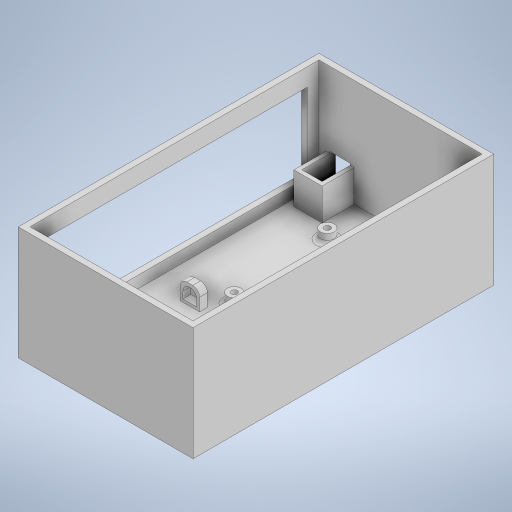
# Autodesk Inventor part: CajaControladora
Saved by Autodesk Inventor 2024 (Build 280153000, 153)
## iProperties
Created: 2023-11-26
Part Number: CajaControladora
Material: Genérico
Document SubType Name: Modeling
Designer: sergi
Density: 1 g/cm^3
Appearance: Valor por defecto
Author: sergi
Autodesk Inventor part; units mm, degrees
ref_plane "YZ Plane" through (0, 0, 0) normal (1, 0, 0) x (0, 1, 0)
ref_plane "XZ Plane" through (0, 0, 0) normal (0, 1, 0) x (-1, 0, 0)
ref_plane "XY Plane" through (0, 0, 0) normal (0, 0, 1) x (1, 0, 0)
sketch "Arduino" plane through (0, 0, 0) normal (0, 1, 0) x (-1, 0, 0)
  line L0 (14.7, 0) -> (48.2, 0)
  line L1 (53.2, -2.5) -> (53.2, -68.5)
  line L2 (0, -2.5) -> (12.2, -2.5)
  line L3 (12.2, -2.5) -> (14.7, 0)
  line L4 (53.2, -2.5) -> (50.7, -2.5)
  line L5 (50.7, -2.5) -> (48.2, 0)
  line L6 (0, -2.5) -> (0, -68.5)
  line L7 (0, -68.5) -> (9.8, -68.5)
  line L8 (9.8, -68.5) -> (9.8, -76.7)
  line L9 (9.8, -76.7) -> (21.92, -76.7)
  line L10 (21.92, -76.7) -> (21.92, -68.5)
  line L11 (21.92, -68.5) -> (41.57, -68.5)
  line L12 (41.57, -68.5) -> (41.57, -73.55)
  line L13 (41.57, -73.55) -> (50.62, -73.55)
  line L14 (50.62, -73.55) -> (50.62, -68.5)
  line L15 (53.2, -68.5) -> (50.62, -68.5)
  line L16 (0, -68.5) -> (9.8, -68.5)
  line L17 (21.92, -68.5) -> (41.57, -68.5)
  line L18 (50.62, -68.5) -> (53.2, -68.5)
  line L19 (0, -2.5) -> (12.2, -2.5)
  line L20 (50.7, -2.5) -> (53.2, -2.5)
  circle A0 centre (18, -2.25) radius 1.575
  circle A1 centre (46.2, -2.25) radius 1.575
  line L21 (53.2, -68.5) -> (53.2, -53.35)
  circle A2 centre (50.88, -54.5) radius 1.575
  circle A3 centre (2.3, -53.5) radius 1.575
  dimension "d4" = 135
  dimension "d5" = 2.5
  dimension "d6" = 135
  dimension "d7" = 66
  dimension "d8" = 9.8
  dimension "d9" = 12.12
  dimension "d10" = 19.65
  dimension "d11" = 5.05
  dimension "d12" = 9.05
  dimension "d15" = 3.15
  dimension "d17" = 3.15
  dimension "d21" = 3.15
  constraints: 44 end point, 15 perpendicular, 4 centre point, 1 horizontal, 1 point on line
  measures "d4" angle of L3 L2
  measures "d5" distance of L1.start L4.end
  measures "d6" angle of L4 L5
  measures "d7" distance of L6.end L2.start
  measures "d8" distance of L6.end L7.end
  measures "d9" distance of L8.end L9.end
  measures "d10" distance of L10.end L11.end
  measures "d11" distance of L11.end L12.end
  measures "d12" distance of L12.end L13.end
  measures "d15" diameter of A0
  measures "d17" diameter of A1
  measures "d21" diameter of A2
sketch "Conector" plane through (0, 0, 0) normal (0, 1, 0) x (-1, 0, 0)
  line L0 (21.92, -68.5) -> (41.57, -68.5) projected
  line L1 (41.57, -73.55) -> (50.62, -73.55) projected
  line L2 (53.2, -2.5) -> (53.2, -68.5) projected
  line L3 (0, -2.5) -> (0, -68.5) projected
  line L4 (0, -68.5) -> (9.8, -68.5) projected
  circle A0 centre (50.88, -54.5) radius 1.575 projected
  line L5 (53.2, -68.5) -> (50.62, -68.5) projected
  line L6 (50.62, -68.5) -> (53.2, -68.5) projected
  line L7 (53.2, -68.5) -> (53.2, -53.35) projected
  line L8 (50.62, -73.55) -> (50.62, -68.5) projected
  circle A1 centre (2.3, -53.5) radius 1.575 projected
  line L9 (21.92, -68.5) -> (41.57, -68.5) projected
  line L10 (0, -68.5) -> (9.8, -68.5) projected
  line L11 (21.92, -76.7) -> (21.92, -68.5) projected
  line L12 (9.8, -68.5) -> (9.8, -76.7) projected
  line L13 (9.8, -76.7) -> (21.92, -76.7) projected
  line L14 (41.57, -68.5) -> (41.57, -73.55) projected
  line L15 (61.92, -76.7) -> (71.32, -76.7)
  line L16 (71.32, -76.7) -> (71.32, -62.9)
  line L17 (71.32, -62.9) -> (61.92, -62.9)
  line L18 (61.92, -62.9) -> (61.92, -76.7)
  point P0 (0, 0)
  dimension "d25" = 40
  dimension "d26" = 9.4
  dimension "d27" = 13.8
  dimension "d28" = 11.3
  constraints: 8 end point, 2 parallel, 1 horizontal, 1 perpendicular
  measures "d25" distance of L11.start L15.start
  measures "d26" distance of L17.end L16.end
  measures "d27" distance of L16.end L15.end
  measures "d28" distance between parallel lines of L8 L18
sketch "PlacaRele" plane through (0, 0, 0) normal (0, 1, 0) x (-1, 0, 0)
  line L0 (0, 0) -> (0, 35)
  line L1 (0, 35) -> (70, 35)
  line L2 (70, 35) -> (70, 65)
  line L3 (70, 65) -> (0, 65)
  line L4 (0, 65) -> (0, 35)
  line L5 (69, 36) -> (1, 36)
  line L6 (1, 36) -> (1, 64)
  line L7 (1, 64) -> (69, 64)
  line L8 (69, 64) -> (69, 36)
  circle A0 centre (2, 37) radius 1
  circle A1 centre (2, 63) radius 1
  circle A2 centre (68, 37) radius 1
  circle A3 centre (68, 63) radius 1
  dimension "d29" = 35
  dimension "d30" = 70
  dimension "d31" = 30
  dimension "d32" = 1
  dimension "d34" = 2
  dimension "d35" = 2
  dimension "d36" = 2
  dimension "d37" = 2
  constraints: 18 end point, 8 tangent, 4 centre point, 4 parallel, 2 perpendicular, 1 horizontal, 1 vertical, 3 other
  measures "d29" distance of L0.start L0.end
  measures "d30" distance of L3.end L2.end
  measures "d31" distance of L2.end L1.end
  measures "d32" distance between parallel lines of L1 L5
  measures "d34" diameter of A0
  measures "d35" diameter of A1
  measures "d36" diameter of A2
  measures "d37" diameter of A3
sketch "Boceto4" plane through (0, 0, 0) normal (0, 1, 0) x (-1, 0, 0)
  line L0 (0, 65) -> (71.32, 65)
  line L1 (71.32, 65) -> (71.32, -76.7)
  line L2 (71.32, -76.7) -> (0, -76.7)
  line L3 (0, -76.7) -> (0, 65)
  line L4 (77.32, -76.7) -> (77.32, 71)
  line L5 (77.32, 71) -> (-6, 71)
  line L6 (-6, 71) -> (-6, -76.7)
  line L7 (80.32, 74) -> (80.32, -76.7)
  line L8 (-9, -76.7) -> (-9, 74)
  line L9 (-9, 74) -> (80.32, 74)
  line L10 (71.32, -62.9) -> (61.92, -62.9)
  line L11 (61.92, -62.9) -> (61.92, -76.7)
  line L12 (61.92, -76.7) -> (71.32, -76.7)
  line L13 (71.32, -76.7) -> (71.32, -62.9)
  line L14 (61.42, -62.4) -> (71.82, -62.4)
  line L15 (71.82, -62.4) -> (71.82, -76.7)
  line L16 (61.42, -76.7) -> (61.42, -62.4)
  line L17 (73.82, -60.4) -> (59.42, -60.4)
  line L18 (59.42, -60.4) -> (59.42, -76.7)
  line L19 (73.82, -76.7) -> (73.82, -60.4)
  line L20 (0, -76.7) -> (-6, -76.7)
  line L21 (71.32, -76.7) -> (77.32, -76.7)
  line L22 (80.32, -76.7) -> (80.32, -79.7)
  line L23 (80.32, -79.7) -> (-9, -79.7)
  line L24 (-9, -79.7) -> (-9, -76.7)
  line L25 (14.7, 0) -> (48.2, 0) projected
  line L26 (53.2, -2.5) -> (53.2, -68.5) projected
  line L27 (0, -2.5) -> (12.2, -2.5) projected
  line L28 (12.2, -2.5) -> (14.7, 0) projected
  line L29 (53.2, -2.5) -> (50.7, -2.5) projected
  line L30 (50.7, -2.5) -> (48.2, 0) projected
  line L31 (0, -2.5) -> (0, -68.5) projected
  line L32 (0, -2.5) -> (12.2, -2.5) projected
  circle A0 centre (18, -2.25) radius 1.575 projected
  circle A1 centre (46.2, -2.25) radius 1.575 projected
  line L33 (50.7, -2.5) -> (53.2, -2.5) projected
  line L34 (0, -68.5) -> (9.8, -68.5) projected
  circle A2 centre (50.88, -54.5) radius 1.575 projected
  line L35 (53.2, -68.5) -> (50.62, -68.5) projected
  line L36 (50.62, -68.5) -> (53.2, -68.5) projected
  line L37 (53.2, -68.5) -> (53.2, -53.35) projected
  line L38 (50.62, -73.55) -> (50.62, -68.5) projected
  line L39 (41.57, -73.55) -> (50.62, -73.55) projected
  circle A3 centre (2.3, -53.5) radius 1.575 projected
  line L40 (21.92, -68.5) -> (41.57, -68.5) projected
  line L41 (21.92, -68.5) -> (41.57, -68.5) projected
  line L42 (0, -68.5) -> (9.8, -68.5) projected
  line L43 (21.92, -76.7) -> (21.92, -68.5) projected
  line L44 (9.8, -68.5) -> (9.8, -76.7) projected
  line L45 (9.8, -76.7) -> (21.92, -76.7) projected
  line L46 (41.57, -68.5) -> (41.57, -73.55) projected
  line L47 (53.2, -68.5) -> (50.62, -68.5) projected
  line L48 (50.62, -68.5) -> (53.2, -68.5) projected
  line L49 (50.62, -73.55) -> (50.62, -68.5) projected
  line L50 (53.2, -68.5) -> (53.2, -53.35) projected
  circle A4 centre (50.88, -54.5) radius 1.575 projected
  line L51 (41.57, -73.55) -> (50.62, -73.55) projected
  line L52 (41.57, -68.5) -> (41.57, -73.55) projected
  line L53 (21.92, -68.5) -> (41.57, -68.5) projected
  line L54 (21.92, -76.7) -> (21.92, -68.5) projected
  line L55 (9.8, -68.5) -> (9.8, -76.7) projected
  line L56 (9.8, -76.7) -> (21.92, -76.7) projected
  line L57 (53.2, -2.5) -> (53.2, -68.5) projected
  line L58 (0, -68.5) -> (9.8, -68.5) projected
  line L59 (0, -68.5) -> (9.8, -68.5) projected
  circle A5 centre (2.3, -53.5) radius 1.575 projected
  line L60 (0, -2.5) -> (0, -68.5) projected
  line L61 (21.92, -68.5) -> (41.57, -68.5) projected
  point P0 (1, 64)
  point P1 (69, 36)
  point P2 (70, 35)
  point P3 (69, 64)
  point P4 (70, 65)
  point P5 (0, 0)
  point P6 (0, 0)
  dimension "d39" = 6
  dimension "d40" = 3
  dimension "d41" = 0.5
  dimension "d42" = 2
  dimension "d43" = 3
  constraints: 50 end point, 8 parallel, 8 perpendicular, 5 point on line, 3 horizontal, 1 vertical
  measures "d39" distance between parallel lines of L1 L4
  measures "d40" distance between parallel lines of L4 L7
  measures "d41" distance between parallel lines of L10 L14
  measures "d42" distance between parallel lines of L14 L17
  measures "d43" distance of L7.end L22.end
sketch "Boceto5" plane through (0, 0, 0) normal (0, 1, 0) x (-1, 0, 0)
  line L0 (-9, 74) -> (80.32, 74) projected
  line L1 (80.32, 74) -> (80.32, -76.7) projected
  line L2 (80.32, -79.7) -> (-9, -79.7) projected
  line L3 (-9, -76.7) -> (-9, 74) projected
  line L4 (-6, 71) -> (-6, -76.7) projected
  line L5 (71.32, -76.7) -> (0, -76.7) projected
  line L6 (0, -76.7) -> (-6, -76.7) projected
  line L7 (71.32, -76.7) -> (77.32, -76.7) projected
  line L8 (77.32, -76.7) -> (77.32, 71) projected
  line L9 (77.32, 71) -> (-6, 71) projected
  line L10 (80.32, -76.7) -> (80.32, -79.7) projected
  line L11 (-9, -79.7) -> (-9, -76.7) projected
  point P0 (0, 0)
extrude "Extrusión1" add sketch "Boceto5" along normal blind 50
sketch "Boceto6" plane through (0, 0, 0) normal (0, -1, 0) x (1, 0, 0)
  line L0 (9, 74) -> (9, -79.7) projected
  line L1 (-80.32, 74) -> (9, 74) projected
  line L2 (-80.32, -79.7) -> (-80.32, 74) projected
  line L3 (9, -79.7) -> (-80.32, -79.7) projected
  line L4 (-77.32, -76.7) -> (6, -76.7) projected
  line L5 (-77.32, 71) -> (-77.32, -76.7) projected
  line L6 (6, 71) -> (-77.32, 71) projected
  line L7 (6, -76.7) -> (6, 71) projected
  point P0 (0, 0)
extrude "Extrusión2" add sketch "Boceto6" along normal blind 5
sketch "Boceto7" plane through (0, -5, 0) normal (0, -1, 0) x (1, 0, 0)
  line L0 (-80.32, -79.7) -> (9, -79.7) projected
  line L1 (-80.32, 74) -> (-80.32, -79.7) projected
  line L2 (9, 74) -> (-80.32, 74) projected
  line L3 (9, -79.7) -> (9, 74) projected
  point P0 (0, 0)
extrude "Extrusión3" add sketch "Boceto7" along normal blind 3
sketch "Boceto10" plane through (-77.32, 50, -76.7) normal (0, 0, 1) x (1, 0, 0)
  line L0 (6, -50) -> (77.32, -50) projected
  line L1 (67.52, -50) -> (67.52, -48.4)
  line L2 (67.52, -48.4) -> (55.4, -48.4)
  line L3 (55.4, -48.4) -> (55.4, -37.7)
  line L4 (55.4, -37.7) -> (67.52, -37.7)
  line L5 (67.52, -37.7) -> (67.52, -48.4)
  line L6 (68.52, -36.7) -> (54.4, -36.7)
  line L7 (54.4, -36.7) -> (54.4, -49.4)
  line L8 (54.4, -49.4) -> (68.52, -49.4)
  line L9 (68.52, -49.4) -> (68.52, -36.7)
  point P0 (77.32, -50)
  point P1 (55.4, -50)
  point P2 (55.4, -50)
  point P3 (55.4, -50)
  point P4 (67.52, -50)
  dimension "d62" = 1.6
  dimension "d63" = 10.7
  dimension "d64" = 1
  constraints: 18 end point, 4 parallel, 2 perpendicular, 1 horizontal, 1 vertical, 4 other
  measures "d62" distance of L1.start L1.end
  measures "d63" distance of L2.end L3.end
  measures "d64" distance between parallel lines of L4 L6
extrude "Extrusión6" cut sketch "Boceto10" against normal blind 10.9 contours L2 L3 L4 L5 | L9 L8 L7 L6
sketch "Boceto8" plane through (0, -5, 0) normal (0, 1, 0) x (1, 0, 0)
  circle A0 centre (-2.3, 53.5) radius 1.575 projected
  circle A1 centre (-18, 2.25) radius 1.575 projected
  line L0 (-73.82, 60.4) -> (-59.42, 60.4) projected
  line L1 (-59.42, 60.4) -> (-59.42, 76.7) projected
  line L2 (-61.42, 62.4) -> (-71.82, 62.4) projected
  line L3 (-61.42, 76.7) -> (-61.42, 62.4) projected
  line L4 (-71.82, 62.4) -> (-71.82, 76.7) projected
  line L5 (-73.82, 76.7) -> (-73.82, 60.4) projected
  line L6 (0, -35) -> (-70, -35) projected
  line L7 (-70, -35) -> (-70, -65) projected
  line L8 (-70, -65) -> (0, -65) projected
  line L9 (0, -65) -> (0, -35) projected
  circle A2 centre (-2, -37) radius 1 projected
  circle A3 centre (-2, -63) radius 1 projected
  circle A4 centre (-68, -37) radius 1 projected
  circle A5 centre (-68, -63) radius 1 projected
  circle A6 centre (-46.2, 2.25) radius 1.575 projected
  circle A7 centre (-50.88, 54.5) radius 1.575 projected
  circle A8 centre (-2.3, 53.5) radius 3.575
  circle A9 centre (-18, 2.25) radius 3.575
  circle A10 centre (-46.2, 2.25) radius 3.575
  circle A11 centre (-50.88, 54.5) radius 3.575
  circle A12 centre (-68, -37) radius 2.5
  circle A13 centre (-68, -63) radius 2.5
  circle A14 centre (-2, -37) radius 2.5
  circle A15 centre (-2, -63) radius 2.5
  point P0 (0, 0)
  dimension "d50" = 2
  dimension "d51" = 2
  dimension "d52" = 2
  dimension "d53" = 2
  dimension "d54" = 1.5
  dimension "d55" = 1.5
  dimension "d56" = 1.5
  dimension "d57" = 1.5
  constraints: 8 centre point
  measures "d50" radial gap between concentric circles of A0 A8
  measures "d51" radial gap between concentric circles of A1 A9
  measures "d52" radial gap between concentric circles of A6 A10
  measures "d53" radial gap between concentric circles of A7 A11
  measures "d54" radial gap between concentric circles of A4 A12
  measures "d55" radial gap between concentric circles of A5 A13
  measures "d56" radial gap between concentric circles of A2 A14
  measures "d57" radial gap between concentric circles of A3 A15
extrude "Extrusión4" add sketch "Boceto8" along normal blind 5 contours A14 L9 L6 | L6 A14 | A14 L9 | A12 L7 L6 | L6 A12 | A15 L9 | L9 A15 L8 | L8 A15 | L7 A12 | A13 L8 | L8 A13 L7 | L7 A13 | A8 | A9 | A10 | A11 picked at (-1.9598, -35.3358) picked at (-67.9598, -35.3358) picked at (-1.9598, -64.6642) picked at (-67.9598, -64.6642)
sketch "Boceto9" plane through (0, -5, 0) normal (0, 1, 0) x (1, 0, 0)
  circle A0 centre (-68, -37) radius 2.5 projected
  circle A1 centre (-18, 2.25) radius 3.575 projected
  circle A2 centre (-46.2, 2.25) radius 3.575 projected
  circle A3 centre (-2, -37) radius 2.5 projected
  circle A4 centre (-68, -63) radius 2.5 projected
  circle A5 centre (-50.88, 54.5) radius 3.575 projected
  circle A6 centre (-2, -63) radius 2.5 projected
  circle A7 centre (-2.3, 53.5) radius 3.575 projected
  line L0 (-77.32, 76.7) -> (-77.32, -71) projected
  line L1 (-77.32, -71) -> (6, -71) projected
  line L2 (6, -71) -> (6, 76.7) projected
  line L3 (6, 76.7) -> (-77.32, 76.7) projected
  line L4 (-73.82, 76.7) -> (-73.82, 60.4) projected
  line L5 (-73.82, 60.4) -> (-59.42, 60.4) projected
  line L6 (-59.42, 60.4) -> (-59.42, 76.7) projected
  line L7 (-61.42, 76.7) -> (-61.42, 62.4) projected
  line L8 (-61.42, 62.4) -> (-71.82, 62.4) projected
  line L9 (-71.82, 62.4) -> (-71.82, 76.7) projected
  point P0 (0, 0)
sketch "Boceto11" plane through (-77.32, 50, -76.7) normal (0, 0, 1) x (1, 0, 0)
  line L0 (68.52, -49.4) -> (54.4, -49.4) projected
  line L1 (15.9, -50) -> (5.5, -50) projected
  line L2 (0, 0) -> (0, -55) projected
  line L3 (54.4, -49.4) -> (0, -49.4)
  line L4 (15.9, -50) -> (15.9, -49.4)
  line L5 (6, -50) -> (0, -50) projected
  line L6 (5.5, -50) -> (5.5, -49.4)
  line L7 (15.9, -49.4) -> (5.5, -49.4)
  line L8 (5.5, -49.4) -> (5.5, -37.7)
  line L9 (5.5, -37.7) -> (15.9, -37.7)
  line L10 (15.9, -37.7) -> (15.9, -49.4)
  point P0 (77.32, -50)
  point P1 (5.5, -50)
  dimension "d67" = 11.7
  constraints: 14 end point, 4 perpendicular, 4 point on line, 2 parallel, 1 horizontal
  measures "d67" distance of L7.end L8.end
extrude "Extrusión7" cut sketch "Boceto11" against normal blind 10.9 contours L3 L8 L9 L10
extrude "Extrusión8" add sketch "Boceto9" along normal up to surface (5.6 mm away) contours L3 L9 L8 L7 L6 L5 L4 | L3 L7 L8 L9
sketch "Boceto12" plane through (-71.82, 0.6, -79.7) normal (0, 1, 0) x (1, 0, 0)
  line L0 (12.4, -19.3) -> (12.4, -3) projected
  line L1 (-2, -19.3) -> (12.4, -19.3) projected
  line L2 (-2, -3) -> (-2, -19.3) projected
  line L3 (10.4, -3) -> (10.4, -17.3)
  line L4 (10.4, -17.3) -> (0, -17.3)
  line L5 (0, -17.3) -> (0, -3)
  line L6 (12.4, -3) -> (-2, -3)
  point P0 (71.82, -79.7)
  constraints: 8 end point, 1 perpendicular, 2 other
extrude "Extrusión9" add sketch "Boceto12" along normal blind 10.7 contours L1 L2 L6 L5 L4 L3 L0
sketch "Boceto13" plane through (0, 50, 0) normal (0, 1, 0) x (1, 0, 0)
  line L0 (9, -74) -> (9, 79.7) projected
  line L1 (9, 79.7) -> (-80.32, 79.7) projected
  line L2 (9, -74) -> (9, 79.7) projected
  line L3 (9, 79.7) -> (-80.32, 79.7) projected
  line L4 (-80.32, 79.7) -> (-80.32, -74) projected
  line L5 (-80.32, -74) -> (9, -74) projected
  line L6 (-77.32, 76.7) -> (6, 76.7) projected
  line L7 (6, 76.7) -> (6, -71) projected
  line L8 (6, -71) -> (-77.32, -71) projected
  line L9 (-77.32, -71) -> (-77.32, 76.7) projected
  line L10 (9, 79.7) -> (-71, 79.7)
  line L11 (-71, 79.7) -> (-71, -0.3)
  line L12 (-71, -0.3) -> (9, -0.3)
  line L13 (9, -0.3) -> (9, 79.7)
  point P0 (0, 0)
  dimension "d74" = 80
  dimension "d75" = 80
  constraints: 8 end point, 2 parallel, 1 horizontal, 1 perpendicular
  measures "d74" distance of L12.end L11.end
  measures "d75" distance of L11.end L10.end
fillet "Empalme1" radius 2 8 edges at (-5.875, -5, -53.5) (-21.575, -5, -2.25) (-49.775, -5, -2.25) (-54.455, -5, -54.5) (-4.5, -5, 37) (-70.5, -5, 37) (-70.5, -5, 63) (-4.5, -5, 63)
sketch "Boceto14" plane through (0, -5, 0) normal (0, 1, 0) x (1, 0, 0)
  circle A0 centre (-18, 2.25) radius 5.575 projected
  line L0 (-18, -3.325) -> (-18, -6.325)
  line L1 (-18, -6.325) -> (9.6696, -6.325)
  line L2 (9.6696, -6.325) -> (-86.9175, -6.325)
  line L3 (0, -35) -> (-70, -35) projected
  circle A1 centre (-68, -63) radius 4.5 projected
  circle A2 centre (-2, -37) radius 4.5 projected
  circle A3 centre (-46.2, 2.25) radius 5.575 projected
  circle A4 centre (-2.3, 53.5) radius 5.575 projected
  line L4 (-73.82, 60.4) -> (-73.82, 76.7) projected
  line L5 (-73.82, 76.7) -> (-77.32, 76.7) projected
  line L6 (-77.32, 76.7) -> (-77.32, -71) projected
  line L7 (-77.32, -71) -> (6, -71) projected
  line L8 (6, -71) -> (6, 76.7) projected
  line L9 (6, 76.7) -> (-59.42, 76.7) projected
  line L10 (-59.42, 76.7) -> (-59.42, 60.4) projected
  line L11 (-59.42, 60.4) -> (-73.82, 60.4) projected
  circle A5 centre (-18, 2.25) radius 5.575 projected
  circle A6 centre (-50.88, 54.5) radius 5.575 projected
  circle A7 centre (-68, -37) radius 4.5 projected
  circle A8 centre (-2, -63) radius 4.5 projected
  line L12 (-9.5756, -35) -> (-9.5756, -32)
  line L13 (-9.5756, -32) -> (-83.4107, -32)
  line L14 (-83.4107, -32) -> (13.4584, -32)
  line L15 (6, -6.325) -> (-4, -6.325)
  line L16 (-4, -6.325) -> (-4, -10.325)
  line L17 (-4, -10.325) -> (-14, -10.325)
  line L18 (-14, -10.325) -> (-14, -6.325)
  line L19 (-14, -32) -> (-14, -28)
  line L20 (-14, -28) -> (-4, -28)
  line L21 (-4, -28) -> (-4, -32)
  line L22 (-71.32, -65) -> (-71.32, 76.7) projected
  line L23 (-71.32, -6.325) -> (-61.32, -6.325)
  line L24 (-61.32, -6.325) -> (-61.32, -10.325)
  line L25 (-61.32, -10.325) -> (-51.32, -10.325)
  line L26 (-51.32, -10.325) -> (-51.32, -6.325)
  line L27 (-71.32, -32) -> (-61.32, -32)
  line L28 (-61.32, -32) -> (-61.32, -28)
  line L29 (-61.32, -28) -> (-51.32, -28)
  line L30 (-51.32, -28) -> (-51.32, -32)
  point P0 (0, 0)
  dimension "d77" = 3
  dimension "d78" = 3
  dimension "d79" = 10
  dimension "d80" = 4
  dimension "d81" = 10
  dimension "d82" = 4
  dimension "d83" = 10
  dimension "d84" = 10
  dimension "d85" = 4
  dimension "d86" = 10
  dimension "d87" = 4
  constraints: 42 end point, 21 point on line, 11 perpendicular, 2 vertical, 1 parallel, 1 vertical alignment, 1 other
  measures "d77" distance of L0.start L0.end
  measures "d78" distance of L12.start L12.end
  measures "d79" distance of L15.start L15.end
  measures "d80" distance of L15.end L16.end
  measures "d81" distance of L16.end L17.end
  measures "d82" distance of L19.start L19.end
  measures "d83" distance of L19.end L20.end
  measures "d84" distance of L23.start L23.end
  measures "d85" distance of L23.end L24.end
  measures "d86" distance of L24.end L25.end
  measures "d87" distance of L27.end L28.end
extrude "Extrusión10" add sketch "Boceto14" along normal blind 10 contours L1 L16 L17 L18 | L26 L25 L24 L2 | L14 L13 L19 L20 L21 | L28 L29 L30 L13
sketch "Boceto15" plane through (-4, -5, 6.325) normal (0, 0, -1) x (-1, 0, 0)
  line L0 (10, 0) -> (0, 0) projected
  line L1 (10, 0) -> (10, 10) projected
  line L2 (0, 10) -> (10, 10) projected
  line L3 (0, 0) -> (0, 10) projected
  line L4 (8.5, 8.5) -> (8.5, 1.5)
  line L5 (8.5, 1.5) -> (1.5, 1.5)
  line L6 (1.5, 1.5) -> (1.5, 8.5)
  line L7 (1.5, 8.5) -> (8.5, 8.5)
  line L8 (57.32, 0) -> (47.32, 0) projected
  line L9 (57.32, 0) -> (57.32, 10) projected
  line L10 (47.32, 10) -> (57.32, 10) projected
  line L11 (47.32, 0) -> (47.32, 10) projected
  line L12 (48.82, 8.5) -> (55.82, 8.5)
  line L13 (55.82, 8.5) -> (55.82, 1.5)
  line L14 (55.82, 1.5) -> (48.82, 1.5)
  line L15 (48.82, 1.5) -> (48.82, 8.5)
  point P0 (-4, 5)
  dimension "d90" = 1.5
  dimension "d91" = 1.5
  constraints: 16 end point, 6 other
  measures "d90" distance between parallel lines of L1 L4
  measures "d91" distance between parallel lines of L11 L15
extrude "Extrusión11" cut sketch "Boceto15" against normal blind 60 contours L4 L5 L6 L7 | L12 L13 L14 L15
fillet "Empalme2" radius 3.5 16 edges at (-52.82, 3.5, 8.325) (-59.82, 3.5, 8.325) (-52.82, 3.5, 30) (-59.82, 3.5, 30) (-5.5, 3.5, 30) (-12.5, 3.5, 30) (-12.5, 3.5, 8.325) (-5.5, 3.5, 8.325) (-4, 5, 8.325) (-4, 5, 30) (-14, 5, 30) (-51.32, 5, 8.325) (-61.32, 5, 8.325) (-61.32, 5, 30) (-51.32, 5, 30) (-14, 5, 8.325)
sketch "Boceto16" plane through (-80.32, 50, -79.7) normal (-1, 0, 0) x (0, 0, 1)
  line L0 (153.7, -58) -> (153.7, 0) projected
  line L1 (0, 0) -> (153.7, 0) projected
  line L2 (0, -58) -> (0, 0) projected
  line L3 (153.7, -58) -> (0, -58) projected
  line L4 (144.7, -9) -> (144.7, -49)
  line L5 (144.7, -49) -> (9, -49)
  line L6 (9, -49) -> (9, -9)
  line L7 (9, -9) -> (144.7, -9)
  point P0 (79.7, -50)
  dimension "d95" = 9
  constraints: 8 end point, 3 other
  measures "d95" distance between parallel lines of L1 L7
extrude "Extrusión12" cut sketch "Boceto16" against normal blind 3 contours L4 L5 L6 L7
